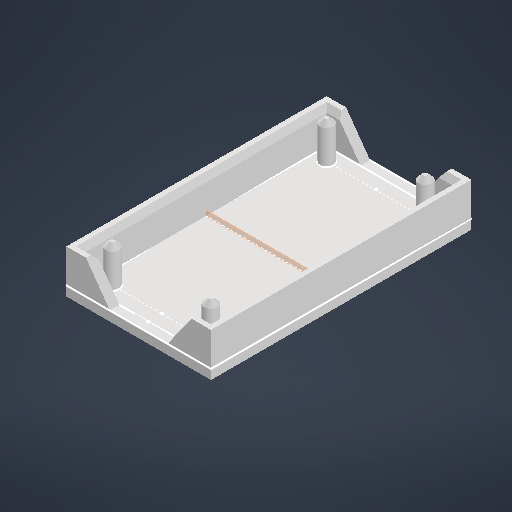
# Autodesk Inventor part: relay board holder
Saved by Autodesk Inventor 2026.2 (Build 302298000, 298)
## iProperties
Created: 2026-01-22
Part Number: relay board holder
Material: Generic
Document SubType Name: Modeling
Designer: User
Density: 1 g/cm^3
Appearance: Default
Author: User
Autodesk Inventor part; units mm, degrees
ref_plane "YZ Plane" through (0, 0, 0) normal (1, 0, 0) x (0, 1, 0)
ref_plane "XZ Plane" through (0, 0, 0) normal (0, 1, 0) x (-1, 0, 0)
ref_plane "XY Plane" through (0, 0, 0) normal (0, 0, 1) x (1, 0, 0)
sketch "Sketch1" plane through (0, 0, 0) normal (0, 1, 0) x (-1, 0, 0)
  line L0 (0, 0) -> (26, 0)
  line L1 (26, 0) -> (26, -50)
  line L2 (26, -50) -> (0, -50)
  line L3 (0, -50) -> (0, 0)
  line L4 (28, 2) -> (-2, 2)
  line L5 (-2, 2) -> (-2, -52)
  line L6 (-2, -52) -> (28, -52)
  line L7 (28, -52) -> (28, 2)
  circle A0 centre (2.775, -2.78) radius 1.4
  circle A1 centre (23.225, -2.78) radius 1.4
  line L8 (2.775, -2.78) -> (23.225, -2.78) construction
  line L9 (26, -25) -> (0, -25) construction
  circle A2 centre (2.775, -47.22) radius 1.4
  circle A3 centre (23.225, -47.22) radius 1.4
  line L10 (2.775, -47.22) -> (23.225, -47.22) construction
  point P0 (13, 0)
  point P1 (13, -2.78)
  point P2 (13, -47.22)
  dimension "d0" = 2
  dimension "d1" = 50
  dimension "d2" = 26
  dimension "d3" = 2.8
  dimension "d4" = 2.8
  dimension "d5" = 23.25
  dimension "d6" = 0
  dimension "d7" = 1.38
  constraints: 22 end point, 4 centre point, 4 midpoint, 4 parallel, 3 symmetric about line, 2 horizontal, 2 perpendicular, 5 other
  measures "d0" distance between parallel lines of L0 L4
  measures "d1" distance of L2.end L0.start
  measures "d2" distance of L0.start L0.end
  measures "d3" diameter of A0
  measures "d4" diameter of A1
  measures "d6" horizontal distance of point (13, 0) point (13, -2.78)
  measures "d7" distance edge to line of A0 L0
extrude "Extrusion1" add sketch "Sketch1" against normal blind 2 contours L0 L1 L2 L3 | L7 L6 L5 L4 | A0 | A1 | A2 | A3
extrude "Extrusion2" add sketch "Sketch1" along normal blind 7 contours L7 L6 L5 L4
extrude "Extrusion3" add sketch "Sketch1" along normal blind 8 contours A0 | A1 | A2 | A3
chamfer "Chamfer1" distance 1 angle 45 8 edges at (-1.375, 8, -2.78) (-21.825, 8, -47.22) (-13, 7, -50) (-26, 7, -25) (0, 7, -25) (-1.375, 8, -47.22) (-21.825, 8, -2.78) (-13, 7, 0)
sketch "Sketch2" plane through (-28, -2, 2) normal (0, 0, 1) x (1, 0, 0)
  line L0 (29, 9) -> (1, 9) projected
  line L1 (28, 2) -> (28, 8) projected
  line L2 (2.0702, 9) -> (28, 9)
  line L3 (28, 9) -> (28, 2)
  line L4 (28, 2) -> (2.0702, 2)
  line L5 (2.0702, 2) -> (2.0702, 9)
  line L6 (25.9502, 9) -> (20.9781, 2)
  line L7 (0, 0) -> (30, 0) projected
  line L8 (15, 0) -> (15, 8)
  line L9 (4.0498, 9) -> (9.0219, 2)
  constraints: 14 end point, 3 point on line, 2 parallel, 2 perpendicular, 2 symmetric about line, 1 horizontal, 1 midpoint
extrude "Extrusion4" cut sketch "Sketch2" against normal blind 2 contours L6 L4 L9 L0
ref_plane "Work Plane1" through (-26, 0, -25) normal (0, 0, 1) x (1, 0, 0)
mirror "Mirror1" about plane through (-26, 0, -25) normal (0, 0, 1) of "Extrusion4"
body "Solid1"
